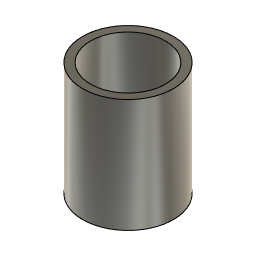
test-fit-inserts (Autodesk Fusion 360 design; units mm, degrees)
Autodesk Fusion 360 part; units mm, degrees
note: some values were not read from the file. Set by a fixed rule: which sketch regions a step uses.
sketch "Esquisse1" plane through (0, 0, 0) normal (0, 0, 1) x (1, 0, 0)
  circle A0 centre (0, 0) radius 4
  circle A1 centre (0, 0) radius 3.2
  circle A2 centre (0, 0) radius 3.3
  circle A3 centre (0, 0) radius 1.6
  line L0 (0, 3.3) -> (-2.8579, 1.65)
  line L1 (-2.8579, 1.65) -> (-2.8579, -1.65)
  line L2 (-2.8579, -1.65) -> (0, -3.3)
  line L3 (0, -3.3) -> (2.8579, -1.65)
  line L4 (2.8579, -1.65) -> (2.8579, 1.65)
  line L5 (2.8579, 1.65) -> (0, 3.3)
  dimension "d2" = 3.2
  dimension "d3" = 6.6
  dimension "d4" = 6.4
  dimension "d5" = 8
  constraint coincident A0.centre A1.centre
  constraint concentric A1 A2
  constraint concentric A2 A3
  constraint coincident A2 L0.start
  measures "d2" diameter of A3
  measures "d3" diameter of A2
  measures "d4" diameter of A1
  measures "d5" diameter of A0
extrude "Extrusion1" add sketch "Esquisse1" along normal blind 10 contours A0 | A1 L4 | A1 A2 L4 | A1 L0 L1 L2 L3 L4 L5 | A1 L4 L5 | A1 L3 L4 | A1 L5 | A1 A2 L5 | A1 A2 L3 | A1 L3 | A1 L0 L5 | A1 A2 L0 | A1 L2 L3 | A1 A2 L2 | A1 L0 | A1 A2 L1 | A1 L0 L1 | A1 L2 | A1 L1 L2 | A1 L1 | A3
extrude "Extrusion2" cut sketch "Esquisse1" along normal blind 15.2 contours A3
sketch "Esquisse2" plane through (0, 0, 0) normal (0, 0, 1) x (1, 0, 0)
extrude "Extrusion3" cut sketch "Esquisse1" along normal blind 2.3 contours A1 L0 L1 L2 L3 L4 L5 | A1 L4 L5 | A1 L3 L4 | A1 L0 L5 | A1 L2 L3 | A1 L0 L1 | A1 L1 L2
extrude "Extrusion4" cut sketch "Esquisse1" along normal blind 7.3 from surface at 4.7 contours A1 L4 | A1 A2 L4 | A1 L0 L1 L2 L3 L4 L5 | A1 L4 L5 | A1 L3 L4 | A1 L5 | A1 A2 L5 | A1 A2 L3 | A1 L3 | A1 L0 L5 | A1 A2 L0 | A1 L2 L3 | A1 A2 L2 | A1 L0 | A1 A2 L1 | A1 L0 L1 | A1 L2 | A1 L1 L2 | A1 L1 | A3
chamfer "Chanfrein1" distance 1 angle 45 1 edges at (-1.4917, -0.5786, 4.7)
